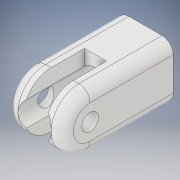
# Autodesk Inventor part: Arm3
Saved by Autodesk Inventor 2017 SP1 (Build 210196100, 196)
## iProperties
Created: 2018-02-11
Part Number: Arm3
Material: ABS Plastic
Document SubType Name: Modeling
Designer: Zach
Density: 1.06 g/cm^3
Appearance: CR White
Author: Zach
Autodesk Inventor part; units mm, degrees
ref_plane "YZ Plane" through (0, 0, 0) normal (1, 0, 0) x (0, 1, 0)
ref_plane "XZ Plane" through (0, 0, 0) normal (0, 1, 0) x (-1, 0, 0)
ref_plane "XY Plane" through (0, 0, 0) normal (0, 0, 1) x (1, 0, 0)
sketch "Sketch1" plane through (0, 0, 0) normal (0, 0, 1) x (1, 0, 0)
  line L0 (0, 0) -> (10, 0)
  line L1 (10, 0) -> (10, 10)
  line L2 (10, 10) -> (0, 10)
  line L3 (0, 10) -> (0, 0)
  dimension "d0" = 10
  dimension "d1" = 10
  constraints: 8 end point, 2 parallel, 1 horizontal, 1 perpendicular
  measures "d0" distance of L2.end L1.end
  measures "d1" distance of L1.end L0.end
extrude "Extrusion1" add sketch "Sketch1" along normal blind 9
sketch "Sketch2" plane through (10, 0, 0) normal (1, 0, 0) x (0, 0, -1)
  circle A0 centre (-15, 5) radius 5 construction
  line L0 (0, 0) -> (0, 10) projected
  arc A1 (-15, 10) -> (-15, 0) centre (-15, 5) ccw
  line L1 (-9, 0) -> (-9, 10) projected
  line L2 (-15, 10) -> (-9, 10)
  line L3 (-15, 0) -> (-9, 0)
  circle A2 centre (-15, 5) radius 1.5
  point P0 (0, 5)
  dimension "d4" = 10
  dimension "d5" = 15
  dimension "d6" = 3
  constraints: 4 end point, 4 point on circle, 3 centre point, 2 horizontal, 1 coincident, 1 concentric, 1 horizontal alignment, 1 midpoint
  measures "d4" diameter of A0
  measures "d5" distance from line of L0 A0.centre
  measures "d6" diameter of A2
extrude "Extrusion2" add sketch "Sketch2" against normal blind 3
sketch "Sketch3" plane through (0, 0, 0) normal (-1, 0, 0) x (0, 0, 1)
  circle A0 centre (15, 5) radius 1.5 projected
  arc A1 (15, 0) -> (15, 10) centre (15, 5) ccw projected
  line L0 (15, 10) -> (9, 10) projected
  line L1 (9, 0) -> (9, 10) projected
  line L2 (9, 0) -> (15, 0) projected
  point P0 (0, 0)
extrude "Extrusion3" add sketch "Sketch3" against normal blind 3
fillet "Fillet1" radius 2 6 edges at (0, 5, 20) (0, 0, 7.5) (0, 10, 7.5) (10, 5, 20) (10, 0, 7.5) (10, 10, 7.5)
sketch "Sketch4" plane through (0, 0, 0) normal (0, 0, -1) x (-1, 0, 0)
  circle A0 centre (-5, 5) radius 1.5
  line L0 (-8, 10) -> (-2, 10) projected
  line L1 (0, 8) -> (0, 2) projected
  point P0 (0, 0)
  point P1 (-5, 10)
  point P2 (0, 5)
  dimension "d12" = 3
  constraints: 2 midpoint, 1 centre point, 1 horizontal alignment, 1 vertical alignment
  measures "d12" diameter of A0
extrude "Extrusion4" cut sketch "Sketch4" against normal through all
ref_plane "Work Plane1" through (0, 0, 3) normal (0, 0, -1) x (-1, 0, 0)
sketch "Sketch5" plane through (0, 0, 3) normal (0, 0, -1) x (-1, 0, 0)
  circle A0 centre (-5, 5) radius 1.5 projected
  circle A1 centre (-5, 5) radius 3
  point P0 (0, 0)
  dimension "d16" = 6
  constraints: 1 centre point, 1 coincident
  measures "d16" diameter of A1
extrude "Extrusion5" cut sketch "Sketch5" against normal through all
sketch "Sketch8" plane through (0, 2, 0) normal (-1, 0, 0) x (0, 0, 1)
  circle A0 centre (15, 3) radius 1.5 projected
  circle A1 centre (15, 3) radius 3
  point P0 (0, -2)
  dimension "d20" = 6
  constraints: 1 centre point, 1 coincident
  measures "d20" diameter of A1
extrude "Extrusion6" cut sketch "Sketch8" against normal blind 1
body "Solid1"
